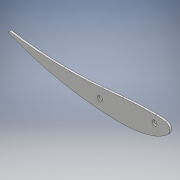
# Autodesk Inventor part: plate
Saved by Autodesk Inventor 2018.2 (Build 222227000, 227)
## iProperties
Created: 2018-03-05
Part Number: plate
Material: 一般
Document SubType Name: Modeling
Designer: ku_sk
Density: 1 g/cm^3
Appearance: 既定
Author: ku_sk
Autodesk Inventor part; units mm, degrees
ref_plane "YZ Plane" through (0, 0, 0) normal (1, 0, 0) x (0, 1, 0)
ref_plane "XZ Plane" through (0, 0, 0) normal (0, 1, 0) x (-1, 0, 0)
ref_plane "XY Plane" through (0, 0, 0) normal (0, 0, 1) x (1, 0, 0)
sketch "スケッチ1" plane through (0, 0, 0) normal (0, 1, 0) x (-1, 0, 0)
  arc A0 (313.7028, 7.555) -> (312.6402, 11.3854) centre (312.9567, 9.4106) ccw projected
  arc A1 (99.4686, -35.9265) -> (313.7028, 7.555) centre (88.5018, 567.6156) ccw projected
  arc A2 (73.7238, -35.6322) -> (99.4686, -35.9265) centre (91.566, 398.982) ccw projected
  arc A3 (26.4399, -27.2272) -> (73.7238, -35.6322) centre (81.048, 142.776) ccw projected
  arc A4 (-0.8557, -13.8205) -> (26.4399, -27.2272) centre (58.458, 72.45) ccw projected
  arc A5 (-8.6045, -6.2961) -> (-0.8557, -13.8205) centre (17.4, 12.732) ccw projected
  arc A6 (-1.8835, 10.4943) -> (-8.6045, -6.2961) centre (0, 0) ccw projected
  arc A7 (18.284, 12.3227) -> (-1.8835, 10.4943) centre (18.66, -103.968) ccw projected
  arc A8 (85.3456, 9.3332) -> (18.284, 12.3227) centre (20.556, -690.396) ccw projected
  arc A9 (85.3456, 9.3332) -> (126.4446, 5.5946) centre (1264.674, 12746.1) ccw projected
  arc A10 (126.4446, 5.5946) -> (203.0985, 2.3771) centre (198.864, 816.2039) ccw projected
  arc A11 (203.0985, 2.3771) -> (312.6402, 11.3854) centre (199.374, 718.188) ccw projected
extrude "押し出し1" add sketch "スケッチ1" along normal blind 4
sketch "スケッチ2" plane through (0, 0, 0) normal (0, -1, 0) x (1, 0, 0)
  circle A0 centre (-20, -2.2582) radius 5
  circle A1 centre (-130, -14.678) radius 5
  line L0 (0, 0) -> (-209.88, -23.6971)
  arc A2 (-313.7028, 7.555) -> (-99.4686, -35.9265) centre (-88.5018, 567.6156) ccw projected
  dimension "d3" = 20
  dimension "d4" = 10
  dimension "d5" = 10
  dimension "d6" = 130
  dimension "d7" = 209.88
  constraints: 2 centre point, 2 end point, 2 point on line, 1 point on circle
  measures "d3" horizontal distance of L0.start A0.centre
  measures "d4" diameter of A0
  measures "d5" diameter of A1
  measures "d6" horizontal distance of L0.start A1.centre
  measures "d7" horizontal distance of L0.start L0.end
extrude "押し出し2" cut sketch "スケッチ2" against normal through all
